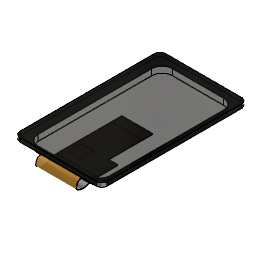
1.47寸触摸屏建模 (Autodesk Fusion 360 design; units mm, degrees)
part number: 2026-01-21-13-45-18-748
Autodesk Fusion 360 part; units mm, degrees
sketch "草图1" plane through (0, 0, 0) normal (0, 0, 1) x (1, 0, 0)
  line L0 (0, 0) -> (23.9, 0)
  line L1 (23.9, 0) -> (23.9, -39.9)
  line L2 (23.9, -39.9) -> (0, -39.9)
  line L3 (0, -39.9) -> (0, 0)
  line L4 (7.7265, 0) -> (7.7265, -1.52) construction
  line L5 (0, -5.5) -> (2.0837, -5.5) construction
  line L6 (2.0837, -5.5) -> (2.0837, 0) construction
  line L7 (7.7265, -1.52) -> (0, -1.52) construction
  line L8 (2.0837, -1.52) -> (21.8337, -1.52)
  line L9 (21.8337, -1.52) -> (21.8337, -38.38)
  line L10 (21.8337, -38.38) -> (2.0837, -38.38)
  line L11 (2.0837, -38.38) -> (2.0837, -1.52)
  line L12 (7.1501, -1.52) -> (7.1501, -2.29) construction
  line L13 (2.0837, -3.1305) -> (2.9264, -3.1305) construction
  line L14 (7.1501, -2.29) -> (2.0837, -2.2916) construction
  line L15 (2.9264, -3.1305) -> (2.9251, -1.52) construction
  line L16 (5.4257, -2.2913) -> (18.4729, -2.2913)
  line L17 (20.9729, -4.7913) -> (20.9729, -33.0233)
  line L18 (18.4729, -35.5233) -> (5.4257, -35.5233)
  line L19 (2.9257, -33.0233) -> (2.9257, -4.7913)
  arc A0 (20.9729, -4.7913) -> (18.4729, -2.2913) centre (18.4729, -4.7913) ccw
  arc A1 (5.4257, -2.2913) -> (2.9257, -4.7913) centre (5.4257, -4.7913) ccw
  arc A2 (18.4729, -35.5233) -> (20.9729, -33.0233) centre (18.4729, -33.0233) ccw
  arc A3 (2.9257, -33.0233) -> (5.4257, -35.5233) centre (5.4257, -33.0233) ccw
  point P0 (2.9257, -2.2913)
  point P1 (20.9729, -2.2913)
  point P2 (2.9257, -35.5233)
  dimension "d13" = 23.9
  dimension "d14" = 39.9
  dimension "d15" = 1.52
  dimension "d16" = 2.0837
  dimension "d17" = 19.75
  dimension "d18" = 36.86
  dimension "d19" = 0.77
  dimension "d20" = 0.8427
  dimension "d21" = 18.0472
  dimension "d22" = 33.232
  dimension "d23" = 2.5
  dimension "d24" = 2.5
  dimension "d25" = 2.5
  dimension "d26" = 2.5
  constraint horizontal L0
  constraint vertical L1
  constraint horizontal L2
  constraint vertical L3
  constraint coincident L0.start L3.end
  constraint coincident L0 L4.start
  constraint perpendicular L0 L4
  constraint coincident L3 L5.start
  constraint perpendicular L3 L5
  constraint coincident L0 L6.end
  constraint perpendicular L0 L6
  constraint coincident L3 L7.end
  constraint perpendicular L3 L7
  constraint horizontal L8
  constraint vertical L9
  constraint horizontal L10
  constraint vertical L11
  constraint coincident L7 L8.start
  constraint coincident L6 L8.start
  constraint coincident L7 L12.start
  constraint perpendicular L7 L12
  constraint coincident L11 L13.start
  constraint perpendicular L11 L13
  constraint coincident L11 L14.end
  constraint coincident L8 L15.end
  constraint horizontal L16
  constraint vertical L17
  constraint horizontal L18
  constraint vertical L19
  constraint coincident L14 P0
  constraint coincident L15 P0
  constraint coincident P1 L16
  constraint coincident P1 L17
  constraint tangent L16 A0
  constraint tangent L17 A0
  constraint coincident P0 L16
  constraint coincident P0 L19
  constraint tangent L16 A1
  constraint tangent L19 A1
  constraint tangent L17 A2
  constraint tangent L18 A2
  constraint coincident P2 L18
  constraint coincident P2 L19
  constraint tangent L18 A3
  constraint tangent L19 A3
  measures "d13" distance of L0.start L0.end
  measures "d14" distance of L0.start L2.end
  measures "d15" distance of L4.start L4.end
  measures "d16" distance of L5.start L5.end
  measures "d17" distance of L8.start L8.end
  measures "d18" distance of L8.start L10.end
  measures "d19" distance of L12.start L12.end
  measures "d20" distance of L13.start L13.end
  measures "d21" distance of P0 P1
  measures "d22" distance of P0 P2
  measures "d23" radius of A0
  measures "d24" radius of A1
  measures "d25" radius of A2
  measures "d26" radius of A3
extrude "拉伸1" add sketch "草图1" along normal blind 1.1 contours L16 L17 L18 L19 A0 A1 A2 A3 makes body 1
extrude "拉伸2" add sketch "草图1" along normal blind 1.1 separate body contours L0 L1 L2 L3 | L8 L9 L10 L11 makes body 2
extrude "拉伸3" add sketch "草图1" against normal blind 1.71 contours L8 L9 L10 L11 | L16 L17 L18 L19 A0 A1 A2 A3 bodies 1 2
fillet "圆角1" radius 2.85 4 edges at (2.0837, -38.38, -0.855) (21.8337, -38.38, -0.855) (2.0837, -1.52, -0.855) (21.8337, -1.52, -0.855) on bodies 1
fillet "圆角2" radius 1.5 4 edges at (23.9, -39.9, 0.55) (23.9, 0, 0.55) (0, -39.9, 0.55) (0, 0, 0.55) on bodies 1 2
ref_plane "工作平面1" through (18.4537, -19.95, -0.855) normal (1, 0, 0) x (0, -1, 0)
sketch "草图2" plane through (18.4537, 0, 0) normal (1, 0, 0) x (0, 1, 0)
  line L0 (-40.0737, 0.279) -> (-41.3337, 0.279) construction
  line L1 (-41.3337, 0.279) -> (-41.3337, -3.821) construction
  spline S0 degree 5 poles (-38.4, -0.1) (-38.6489, -0.1241) (-39.1066, -0.1572) (-39.6727, -0.1622) (-40.2067, -0.109) (-40.6122, -0.0856) (-40.8776, -0.2486) (-41.0923, -0.6505) (-41.2846, -1.212) (-41.3379, -1.5449) (-41.3206, -1.6651) (-41.3382, -1.7439) (-41.3415, -1.9119) (-41.1691, -2.142) (-40.7884, -2.3881) (-40.2158, -2.5782) (-39.5476, -2.6559) (-38.9632, -2.6102) (-38.484, -2.4652) (-38.0486, -2.2648) (-37.5389, -2.0636) (-36.9662, -1.9445) (-36.3943, -1.8972) (-35.9431, -1.8867) (-35.7, -1.8867) knots 0 0 0 0 0 0 0.05 0.1 0.15 0.2 0.25 0.3 0.35 0.4 0.45 0.5 0.55 0.6 0.65 0.7 0.75 0.8 0.85 0.9 0.95 1 1 1 1 1 1
  line L2 (-40.9429, -0.2435) -> (-41.4268, -1.6476)
  line L3 (-37, -1.8867) -> (-34.4, -1.8867)
  line L4 (-38.4, -1.7) -> (-30.02, -1.7) construction
  line L5 (-35.7, -1.8867) -> (-30, -1.8867)
  line L6 (-40.7, -2.5) -> (-39.1, -2.7)
  line L7 (-41.3337, -1.521) -> (-41.3337, -2.021)
  line L8 (-36.7517, 0.0593) -> (-40.0483, -0.2593)
  spline S1 degree 3 poles (-38.4115, 0.0194) (-39.4337, -0.0793) (-39.9937, 0.0125) (-40.379, 0.0085) (-40.675, 0.0054) (-40.9025, -0.1183) (-41.0589, -0.3717) (-41.2375, -0.6611) (-41.3747, -1.1063) (-41.4209, -1.3536) (-41.4615, -1.5709) (-41.4457, -1.6334) (-41.4503, -1.6981) (-41.4558, -1.7768) (-41.4586, -1.9894) (-41.2464, -2.1914) (-41.0101, -2.4164) (-40.5136, -2.6385) (-39.9494, -2.7146) (-39.4192, -2.7861) (-38.9191, -2.7237) (-38.5229, -2.5886) (-37.963, -2.3978) (-37.5596, -2.1121) (-36.4532, -2.0315) (-36.2299, -2.0152) (-35.9794, -2.0067) (-35.7, -2.0067) knots 0 0 0 0 0.124236 0.124236 0.124236 0.219713 0.219713 0.219713 0.328762 0.328762 0.328762 0.424581 0.424581 0.424581 0.541088 0.541088 0.541088 0.670846 0.670846 0.670846 0.792816 0.792816 0.792816 0.965215 0.965215 0.965215 1 1 1 1
  line L9 (-35.7, -2.0067) -> (-30, -2.0067)
  line L10 (-38.4, -0.1) -> (-38.3802, -0.1)
  line L11 (-38.3802, 0.0197) -> (-38.4115, 0.0194)
  line L12 (-38.3802, -0.1) -> (-38.3802, 0.0197)
  line L13 (-30, -2.0067) -> (-30, -1.8867)
  point P0 (-41.1848, -0.9456)
  point P1 (-41.3337, -1.771)
  point P2 (-39.9, -2.6)
  dimension "d38" = 1.26
  dimension "d39" = 8.38
  dimension "d40" = 0.12
  constraint horizontal L0
  constraint perpendicular L0 L1
  constraint midpoint P0 L2
  constraint midpoint S0.end L3
  constraint horizontal L4
  constraint parallel L4 L5
  constraint midpoint P2 L6
  constraint midpoint P1 L7
  constraint midpoint L1 P1
  constraint coincident L1 L7.start
  constraint midpoint S0.start L8
  constraint horizontal L10
  constraint vertical L12
  constraint perpendicular L5 L13
  measures "d38" distance of L0.start L0.end
  measures "d39" distance of L4.start L4.end
extrude "拉伸4" add sketch "草图2" against normal blind 11.11 bodies 1
sketch "草图3" plane through (0, 0, -2.0067) normal (0, 0, -1) x (1, 0, 0)
  line L0 (18.4537, 30) -> (18.4537, 35.7)
  line L1 (18.4537, 35.7) -> (7.3437, 35.7)
  line L2 (7.3437, 35.7) -> (7.3437, 30)
  line L3 (7.3437, 30) -> (18.4537, 30)
  line L4 (5.7336, 38.371) -> (5.7336, 33.471) construction
  line L5 (5.7336, 33.471) -> (22, 33.471) construction
  line L6 (8.3624, 33.471) -> (11.8624, 33.471)
  line L7 (11.8624, 33.471) -> (11.8624, 29.971)
  line L8 (11.8624, 29.971) -> (8.3624, 29.971)
  line L9 (8.3624, 29.971) -> (8.3624, 33.471)
  line L10 (7.3437, 30) -> (15.8337, 30)
  line L11 (15.8337, 30) -> (15.8337, 17.83)
  line L12 (15.8337, 17.83) -> (7.3437, 17.83)
  line L13 (7.3437, 17.83) -> (7.3437, 30)
  line L14 (15.8337, 17.83) -> (7.3437, 17.83)
  line L15 (7.3437, 17.83) -> (7.3437, 20.73)
  line L16 (7.3437, 20.73) -> (15.8337, 20.73)
  line L17 (15.8337, 20.73) -> (15.8337, 17.83)
  line L18 (15.7337, 17.93) -> (7.4437, 17.93)
  line L19 (7.4437, 17.93) -> (7.4437, 20.63)
  line L20 (7.4437, 20.63) -> (15.7337, 20.63)
  line L21 (15.7337, 20.63) -> (15.7337, 17.93)
  dimension "d43" = 4.9
  dimension "d44" = 3.5
  dimension "d45" = 3.5
  dimension "d48" = 8.49
  dimension "d49" = 12.17
  dimension "d52" = 2.9
  dimension "d53" = 0.1
  constraint vertical L4
  constraint perpendicular L0 L5
  constraint horizontal L6
  constraint vertical L7
  constraint horizontal L8
  constraint vertical L9
  constraint coincident L5 L6.start
  constraint horizontal L10
  constraint vertical L11
  constraint horizontal L12
  constraint vertical L13
  constraint coincident L2.end L3.start
  constraint horizontal L14
  constraint vertical L15
  constraint horizontal L16
  constraint vertical L17
  measures "d43" distance of L4.start L4.end
  measures "d44" distance of L6.start L6.end
  measures "d45" distance of L6.start L8.end
  measures "d48" distance of L2.end L10.end
  measures "d49" distance of L2.end L12.end
  measures "d52" distance of L11.end L16.end
extrude "拉伸5" add sketch "草图3" along normal blind 1.1 contours L3 L6 L7 L9 L10 bodies 1
extrude "拉伸6" add sketch "草图3" against normal blind 0.12 contours L3 L7 L8 L9 L10 L11 L13 L16 | L11 L12 L13 L14 L15 L16 L17 | L18 L19 L20 L21 bodies 1
extrude "拉伸7" add sketch "草图3" along normal blind 0.1 contours L18 L19 L20 L21 bodies 1
equation "d31 = -2.81 mm + 1.1 mm"
